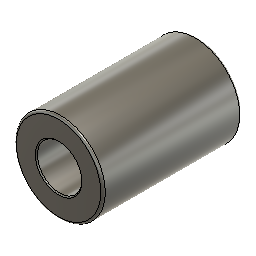
Brass bush, H=25mm (Autodesk Fusion 360 design; units mm, degrees)
Autodesk Fusion 360 part; units mm, degrees
sketch "Sketch1" plane through (0, 0, 0) normal (0, 0, 1) x (1, 0, 0)
  circle A0 centre (0, 0) radius 8
  circle A1 centre (0, 0) radius 4
  dimension "d1" = 8
  dimension "d2" = 16
  constraint coincident A0.centre A1.centre
  measures "d1" diameter of A1
  measures "d2" diameter of A0
extrude "Extrude1" add sketch "Sketch1" along normal blind 25 makes body 1
fillet "Fillet1" radius 0.2 2 edges at (-3.7293, 1.4465, 25) (-3.7293, 1.4465, 0) on bodies 1
fillet "Fillet2" radius 0.4 2 edges at (-7.4586, -2.8929, 25) (-7.4586, -2.8929, 0) on bodies 1
copy_body "Body->Comp1" bodies 1 removing the originals makes body 2 in component "Component"
component "Component" placed x (1, 0, 0) y (0, 1, 0) z (0, 0, 1) at (0, 0, 0)
